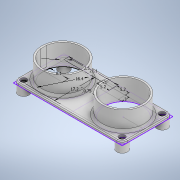
# Autodesk Inventor part: ultrasonic outer cover plate
Saved by Autodesk Inventor 2022 (Build 260153000, 153)
## iProperties
Created: 2022-04-06
Part Number: ultrasonic outer cover plate
Material: Generic
Document SubType Name: Modeling
Designer: a-dubs
Density: 1 g/cm^3
Appearance: Default
Author: a-dubs
Autodesk Inventor part; units mm, degrees
ref_plane "YZ Plane" through (0, 0, 0) normal (1, 0, 0) x (0, 1, 0)
ref_plane "XZ Plane" through (0, 0, 0) normal (0, 1, 0) x (-1, 0, 0)
ref_plane "XY Plane" through (0, 0, 0) normal (0, 0, 1) x (1, 0, 0)
sketch "Sketch1" plane through (0, 0, 0) normal (0, 1, 0) x (-1, 0, 0)
  line L0 (0, 0) -> (0, -17.2)
  circle A0 centre (0, -17.2) radius 1.25
  line L1 (0, -8.6) -> (-8.1, -8.6)
  circle A1 centre (-8.1, -8.6) radius 8.2
  circle A2 centre (0, 0) radius 1.25
  line L2 (1.25, -17.2) -> (2.25, -17.2)
  line L3 (0, -18.45) -> (0, -19.45)
  line L4 (0, -19.45) -> (2.25, -19.45)
  line L5 (2.25, -19.45) -> (2.25, -17.2)
  line L6 (0, -17.2) -> (-21.1, -17.2)
  line L7 (0, 0) -> (-21.1, 0)
  line L8 (0, 1.25) -> (0, 2.25)
  line L9 (1.25, 0) -> (2.25, 0)
  line L10 (2.25, 0) -> (2.25, -17.2)
  line L11 (0, 2.25) -> (2.25, 2.25)
  line L12 (2.25, 2.25) -> (2.25, 0)
  line L13 (0, -19.45) -> (-21.1, -19.45)
  line L14 (0, 2.25) -> (-21.1, 2.25)
  circle A3 centre (0, -17.2) radius 2.25
  circle A4 centre (0, 0) radius 2.25
  line L15 (-21.1, -19.45) -> (-21.1, 2.25)
  line L16 (-42.2, 0) -> (-42.2, -17.2)
  circle A5 centre (-42.2, -17.2) radius 1.25
  line L17 (-42.2, -8.6) -> (-34.1, -8.6)
  circle A6 centre (-34.1, -8.6) radius 8.2
  circle A7 centre (-42.2, 0) radius 1.25
  line L18 (-43.45, -17.2) -> (-44.45, -17.2)
  line L19 (-42.2, -18.45) -> (-42.2, -19.45)
  line L20 (-42.2, -19.45) -> (-44.45, -19.45)
  line L21 (-44.45, -19.45) -> (-44.45, -17.2)
  line L22 (-42.2, -17.2) -> (-21.1, -17.2)
  line L23 (-42.2, 0) -> (-21.1, 0)
  line L24 (-42.2, 1.25) -> (-42.2, 2.25)
  line L25 (-43.45, 0) -> (-44.45, 0)
  line L26 (-44.45, 0) -> (-44.45, -17.2)
  line L27 (-42.2, 2.25) -> (-44.45, 2.25)
  line L28 (-44.45, 2.25) -> (-44.45, 0)
  line L29 (-42.2, -19.45) -> (-21.1, -19.45)
  line L30 (-42.2, 2.25) -> (-21.1, 2.25)
  circle A8 centre (-42.2, -17.2) radius 2.25
  circle A9 centre (-42.2, 0) radius 2.25
  line L31 (-21.1, -17.2) -> (-15.9, -17.2)
  line L32 (-21.1, -17.2) -> (-26.3, -17.2)
  line L33 (-15.9, -17.2) -> (-15.9, -18.2)
  line L34 (-15.9, -18.2) -> (-26.3, -18.2)
  line L35 (-26.3, -18.2) -> (-26.3, -17.2)
  line L36 (-26.3, -17.2) -> (-26.3, -14.2)
  line L37 (-26.3, -14.2) -> (-15.9, -14.2)
  line L38 (-15.9, -14.2) -> (-15.9, -18.2)
  line L39 (-16.3, -8.6) -> (-17.05, -8.6)
  circle A10 centre (-8.1, -8.6) radius 8.95
  line L40 (-25.9, -8.6) -> (-25.15, -8.6)
  circle A11 centre (-34.1, -8.6) radius 8.95
  point P0 (-42.2, -7.3233)
  point P1 (-42.2, -9.8767)
  point P2 (0, -7.3233)
  point P3 (0, -9.8767)
  dimension "d4" = 16.4
  dimension "d0" = 17.2
  dimension "d2" = 2.5
  dimension "d3" = 8.1
  dimension "d7" = 21.1
  dimension "d14" = 5.2
  dimension "d15" = 5.2
  dimension "d16" = 1
  dimension "d17" = 3
  dimension "d21" = 0.75
  constraints: 82 end point, 22 symmetric about line, 11 coincident, 9 perpendicular, 9 vertical, 8 horizontal, 8 point on circle, 5 centre point, 4 horizontal alignment, 4 point on line, 3 parallel, 2 vertical alignment, 1 equal radius, 1 midpoint, 18 other
  measures "d0" distance of L0.start L0.end
  measures "d2" diameter of A0
  measures "d3" distance of L1.start L1.end
  measures "d7" distance of L6.start L6.end
  measures "d14" distance of L6.end L31.end
  measures "d15" distance of L6.end L32.end
  measures "d16" distance of L31.end L33.end
  measures "d17" distance of L32.end L36.end
  measures "d21" distance of L39.start L39.end
extrude "Extrusion1" add sketch "Sketch1" along normal blind 1 contours A2 L9 A4 L0 | L0 A4 L7 A2 | L7 A4 L8 A2 | A4 L10 A3 L0 A10 | L0 A10 L7 A4 | A2 L8 A4 L9 | L7 A10 L15 L14 A4 | A10 L0 A1 | L0 A1 L39 A10 L7 | A4 L11 L12 | L7 A10 | A3 L3 A0 L2 | L5 L4 A3 | L2 A0 L0 A3 | L15 L23 A11 A9 L30 | A10 L6 L38 L37 L15 L7 | A1 L0 A10 L6 L39 | L0 A3 L6 A10 | A3 L6 A0 L3 | L13 L15 L34 L33 L6 A10 A3 | L0 A0 L6 A3 | L15 L37 L36 L22 A11 L23 | A9 L23 A7 L24 | A9 L28 L27 | L24 A7 L25 A9 | A10 L6 | L29 A8 L22 A11 L35 L34 L15 | L37 L38 L6 L15 | L15 L22 L36 L37 | A11 L40 A6 L16 L23 | L23 A11 | A9 L16 A7 L23 | L23 A11 L16 A9 | A9 L16 A11 A8 L26 | L25 A7 L16 A9 | L34 L35 L22 L15 | L15 L6 L33 L34 | A8 L18 A5 L19 | L20 L21 A8 | L19 A5 L22 A8 | A11 L22 L16 A6 L40 | A8 L16 A5 L18 | A8 L16 A11 L22 | L22 A5 L16 A8 | L16 A6 A11 | A11 L22
extrude "Extrusion2" add sketch "Sketch1" against normal blind 3.5 contours A2 L9 A4 L0 | L0 A4 L7 A2 | L7 A4 L8 A2 | A2 L8 A4 L9 | A3 L3 A0 L2 | L2 A0 L0 A3 | A3 L6 A0 L3 | L0 A0 L6 A3 | A9 L23 A7 L24 | L24 A7 L25 A9 | A9 L16 A7 L23 | L25 A7 L16 A9 | A8 L18 A5 L19 | L19 A5 L22 A8 | A8 L16 A5 L18 | L22 A5 L16 A8
fillet "Fillet1" radius 2.25 4 edges at (-2.25, 0.5, 2.25) (-2.25, 0.5, -19.45) (44.45, 0.5, -19.45) (44.45, 0.5, 2.25)
fillet "Fillet2" [suppressed]
fillet "Fillet3" radius 0.4 8 edges at (-1.591, 1, -18.791) (-2.25, 1, -8.6) (-1.591, 1, 1.591) (21.1, 1, 2.25) (43.791, 1, 1.591) (44.45, 1, -8.6) (43.791, 1, -18.791) (21.1, 1, -19.45)
extrude "Extrusion3" add sketch "Sketch1" along normal blind 8 from surface at 1 contours A10 L0 A1 | L0 A1 L39 A10 L7 | L7 A10 | A1 L0 | A1 L0 A10 L6 L39 | A10 L6 | A11 L40 A6 L16 L23 | L23 A11 | A11 L22 L16 A6 L40 | L16 A6 A11 | A11 L22 | L16 A6 picked at (0.0185, -9.3099) picked at (-42.2296, -8.0321)
chamfer "Chamfer1" distance 1 angle 45 2 edges at (43.05, 1, -8.6) (17.05, 1, -8.6)
body "Solid1"
